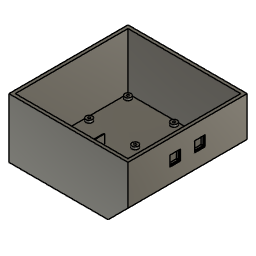
WeatherBox (Autodesk Fusion 360 design; units mm, degrees)
Autodesk Fusion 360 part; units mm, degrees
note: some values were not read from the file. Set by a fixed rule: which face or edge a step refers to.
sketch "Enclosure" plane through (0, 0, 0) normal (0, 0, 1) x (1, 0, 0)
  line L0 (0, 0) -> (150, 0)
  line L1 (150, 0) -> (150, 150)
  line L2 (150, 150) -> (0, 150)
  line L3 (0, 150) -> (0, 0)
  dimension "d1" = 150
  dimension "d2" = 150
  constraint horizontal L0
  constraint vertical L1
  constraint horizontal L2
  constraint vertical L3
  constraint coincident L0.start L3.end
  measures "d1" distance of L0.start L0.end
  measures "d2" distance of L0.start L2.end
extrude "Extrude1" add sketch "Enclosure" along normal blind 75 makes body 1
chamfer "Chamfer1" distance 25 angle 45 1 edges at (150, 75, 0) on bodies 1
shell "Shell1" thickness 4 removed faces 1 at (50, 100, 75) on bodies 1
sketch "Pi Mount" plane through (0, 0, 4) normal (0, 0, 1) x (-1, 0, 0)
  line L0 (-4, -146) -> (-4, -4)
  line L1 (-4, -4) -> (-123.3431, -4)
  line L2 (-123.3431, -146) -> (-4, -146)
  circle A0 centre (-9, -141) radius 4
  line L3 (-123.3431, -4) -> (-123.3431, -146)
  dimension "d13" = 8
  dimension "d39" = 5
  dimension "d40" = 5
  measures "d13" diameter of A0
  measures "d39" distance of L2 A0.centre
  measures "d40" distance of L0 A0.centre
extrude "Extrude2" add sketch "Pi Mount" along normal blind 3.1 contours A0 bodies 1
hole "Hole2" at (9, 141, 7.1) direction (0, 0, -1) diameter 2.9 depth 3.1 tip angle 180 bodies 1
pattern_linear "R-Pattern1" count 2 spacing 58 along (1, 0, 0) count 2 spacing 49 along (0, -1, 0) of "Extrude2", "Hole2"
sketch "Camera Holes" plane through (150, 0, 0) normal (1, 0, 0) x (0, 1, 0)
  line L0 (150, 25) -> (150, 75)
  line L1 (150, 75) -> (0, 75)
  line L2 (0, 75) -> (0, 25)
  line L3 (65, 44.45) -> (53.9, 44.45)
  line L4 (53.9, 44.45) -> (53.9, 55.55)
  line L5 (53.9, 55.55) -> (65, 55.55)
  line L6 (65, 55.55) -> (65, 44.45)
  line L7 (65, 44.45) -> (53.9, 55.55) construction
  line L8 (53.9, 44.45) -> (65, 55.55) construction
  line L9 (0, 50) -> (150, 50) construction
  line L10 (75, 75) -> (75, 0) construction
  line L11 (96.1, 44.45) -> (85, 55.55) construction
  line L12 (85, 44.45) -> (96.1, 55.55) construction
  line L13 (85, 44.45) -> (85, 55.55)
  line L14 (85, 55.55) -> (96.1, 55.55)
  line L15 (96.1, 55.55) -> (96.1, 44.45)
  line L16 (96.1, 44.45) -> (85, 44.45)
  line L17 (66, 43.45) -> (52.9, 43.45)
  line L18 (52.9, 43.45) -> (52.9, 56.55)
  line L19 (52.9, 56.55) -> (66, 56.55)
  line L20 (66, 56.55) -> (66, 43.45)
  line L21 (97.1, 43.45) -> (84, 43.45)
  line L22 (84, 43.45) -> (84, 56.55)
  line L23 (84, 56.55) -> (97.1, 56.55)
  line L24 (97.1, 56.55) -> (97.1, 43.45)
  line L25 (0, 25) -> (150, 25)
  point P0 (59.45, 50)
  point P1 (90.55, 50)
  dimension "d92" = 11.1
  dimension "d93" = 11.1
  dimension "d168" = 11.1
  dimension "d169" = 11.1
  dimension "d170" = 20
  dimension "d177" = -1
  dimension "d178" = -1
  constraint horizontal L3
  constraint perpendicular L3 L4
  constraint parallel L3 L5
  constraint parallel L4 L6
  constraint coincident L7 P0
  constraint coincident L8 P0
  constraint midpoint L2 L9.start
  constraint midpoint L0 L9.end
  constraint coincident P0 L9
  constraint midpoint L1 L10.start
  constraint horizontal L16
  constraint perpendicular L13 L16
  constraint parallel L14 L16
  constraint parallel L13 L15
  constraint coincident P1 L11
  constraint coincident P1 L12
  constraint symmetric L6 L10 L13
  constraint collinear L19 L23
  measures "d92" distance of L4.end L5.end
  measures "d93" distance of L3.end L4.end
  measures "d168" distance of L12.end L11.end
  measures "d169" distance of L12.start L11.end
  measures "d170" distance of L6 L13
extrude "Extrude6" cut sketch "Camera Holes" against normal up to surface (4 mm away) contours L3 L4 L5 L6 | L13 L14 L15 L16 bodies 1
extrude "Extrude10" cut sketch "Camera Holes" against normal blind 1.5875 contours L17 L18 L19 L20 | L21 L22 L23 L24 bodies 1
sketch "Camera Mounts" plane through (146, 0, 0) normal (-1, 0, 0) x (0, -1, 0)
  line L0 (-65, 44.45) -> (-65, 55.55)
  line L1 (-65, 55.55) -> (-53.9, 55.55)
  line L2 (-53.9, 55.55) -> (-53.9, 44.45)
  line L3 (-53.9, 44.45) -> (-65, 44.45)
  line L4 (-4, 26.6569) -> (-4, 75)
  line L5 (-4, 75) -> (-146, 75)
  line L6 (-146, 75) -> (-146, 26.6569)
  line L7 (-69.95, 62.6) -> (-48.95, 62.6) construction
  line L8 (-48.95, 62.6) -> (-48.95, 50.1) construction
  line L9 (-48.95, 50.1) -> (-69.95, 50.1) construction
  line L10 (-69.95, 50.1) -> (-69.95, 62.6) construction
  line L11 (-59.45, 55.55) -> (-59.45, 50) construction
  line L12 (-59.45, 50) -> (-53.9, 50) construction
  line L13 (-85, 44.45) -> (-96.1, 44.45)
  line L14 (-96.1, 44.45) -> (-96.1, 55.55)
  line L15 (-96.1, 55.55) -> (-85, 55.55)
  line L16 (-85, 55.55) -> (-85, 44.45)
  line L17 (-101.05, 62.6) -> (-80.05, 62.6) construction
  line L18 (-101.05, 50.1) -> (-101.05, 62.6) construction
  line L19 (-80.05, 50.1) -> (-101.05, 50.1) construction
  line L20 (-80.05, 62.6) -> (-80.05, 50.1) construction
  line L21 (-85, 50) -> (-90.55, 50) construction
  line L22 (-90.55, 50) -> (-90.55, 55.55) construction
  line L23 (-146, 26.6569) -> (-4, 26.6569)
  dimension "d131" = 21
  dimension "d132" = 12.5
  dimension "d173" = 21
  dimension "d174" = 12.5
  dimension "d176" = 0.1
  constraint horizontal L7
  constraint vertical L8
  constraint horizontal L9
  constraint vertical L10
  constraint midpoint L1 L11.start
  constraint perpendicular L1 L11
  constraint midpoint L2 L12.end
  constraint perpendicular L2 L12
  constraint horizontal L17
  constraint vertical L20
  constraint horizontal L19
  constraint vertical L18
  constraint midpoint L16 L21.start
  constraint midpoint L15 L22.end
  constraint perpendicular L15 L22
  constraint symmetric L18 L20 L22
  constraint collinear L9 L19
  measures "d131" distance of L7.start L7.end
  measures "d132" distance of L7.start L9.end
  measures "d173" distance of L17.start L17.end
  measures "d174" distance of L17.start L18.start
  measures "d176" distance of L19 L21
hole "Hole7" at (146, 48.95, 62.6) at (146, 69.95, 50.1) at (146, 80.05, 62.6) at (146, 101.05, 62.6) at (146, 101.05, 50.1) at (146, 80.05, 50.1) at (146, 69.95, 62.6) at (146, 48.95, 50.1) direction (1, 0, 0) diameter 2.9 depth 2 tip angle 180 bodies 1
sketch "Camera Posts" plane through (146, 0, 0) normal (-1, 0, 0) x (0, -1, 0)
  circle A0 centre (-101.05, 50.1) radius 1.45
  circle A1 centre (-80.05, 62.6) radius 1.45
  circle A2 centre (-48.95, 50.1) radius 1.45
  circle A3 centre (-69.95, 62.6) radius 1.45
  circle A4 centre (-48.95, 62.6) radius 1.45
  circle A5 centre (-69.95, 50.1) radius 1.45
  circle A6 centre (-101.05, 62.6) radius 1.45
  circle A7 centre (-80.05, 50.1) radius 1.45
  line L0 (-65, 44.45) -> (-65, 55.55)
  line L1 (-65, 55.55) -> (-53.9, 55.55)
  line L2 (-53.9, 55.55) -> (-53.9, 44.45)
  line L3 (-53.9, 44.45) -> (-65, 44.45)
  line L4 (-85, 44.45) -> (-96.1, 44.45)
  line L5 (-96.1, 44.45) -> (-96.1, 55.55)
  line L6 (-96.1, 55.55) -> (-85, 55.55)
  line L7 (-85, 55.55) -> (-85, 44.45)
  line L8 (-4, 26.6569) -> (-4, 75)
  line L9 (-4, 75) -> (-146, 75)
  line L10 (-146, 75) -> (-146, 26.6569)
  circle A8 centre (-101.05, 62.6) radius 3.95
  circle A9 centre (-80.05, 62.6) radius 3.95
  circle A10 centre (-101.05, 50.1) radius 3.95
  circle A11 centre (-80.05, 50.1) radius 3.95
  circle A12 centre (-69.95, 62.6) radius 3.95
  circle A13 centre (-48.95, 62.6) radius 3.95
  circle A14 centre (-48.95, 50.1) radius 3.95
  circle A15 centre (-69.95, 50.1) radius 3.95
  line L11 (-146, 26.6569) -> (-4, 26.6569)
  dimension "d193" = 2.5
  constraint equal A8 A10
  constraint equal A8 A11
  constraint equal A8 A9
  constraint equal A8 A12
  constraint equal A8 A15
  constraint equal A8 A14
  constraint equal A8 A13
extrude "Extrude11" add sketch "Camera Posts" along normal blind 7 contours A8 | A9 | A10 | A11 | A12 | A13 | A14 | A15 bodies 1
sketch "SPS30 Mount" plane through (0, 4, 0) normal (0, 1, 0) x (-1, 0, 0)
  line L0 (-4, 75) -> (-146, 75)
  line L1 (-123.3431, 4) -> (-4, 4)
  line L2 (-130, 64) -> (-83.15, 64)
  line L3 (-83.15, 64) -> (-83.15, 17.15)
  line L4 (-83.15, 17.15) -> (-130, 17.15)
  line L5 (-130, 17.15) -> (-130, 64)
  line L6 (-82.15, 16.15) -> (-131, 16.15)
  line L7 (-131, 16.15) -> (-131, 65)
  line L8 (-131, 65) -> (-82.15, 65)
  line L9 (-82.15, 65) -> (-82.15, 16.15)
  line L10 (-103.15, 17.15) -> (-103.15, 16.15)
  line L11 (-130, 17.15) -> (-130, 16.15)
  line L12 (-85.15, 64) -> (-85.15, 65)
  line L13 (-125, 64) -> (-125, 65)
  line L14 (-139.7177, 40.575) -> (-2.7177, 40.575) construction
  line L15 (-106.575, 64) -> (-106.575, 17.15) construction
  line L16 (-130, 40.575) -> (-83.15, 40.575) construction
  line L17 (-4, 4) -> (-4, 75)
  line L18 (-146, 75) -> (-146, 26.6569)
  line L19 (-104.15, 64) -> (-104.15, 75)
  line L20 (-104.15, 75) -> (-103.15, 75)
  line L21 (-103.15, 75) -> (-103.15, 64)
  line L22 (-104.15, 64) -> (-103.15, 64)
  line L23 (-78.15, 40.575) -> (-135, 40.575) construction
  circle A0 centre (-78.15, 40.575) radius 2.35
  circle A1 centre (-135, 40.575) radius 2.35
  circle A2 centre (-135, 40.575) radius 4.85
  circle A3 centre (-78.15, 40.575) radius 4.85
  line L24 (-78.15, 45.425) -> (-135, 45.425)
  line L25 (-135, 35.725) -> (-78.15, 35.725)
  line L26 (-146, 26.6569) -> (-123.3431, 4)
  dimension "d118" = 46.85
  dimension "d119" = 46.85
  dimension "d121" = -1
  dimension "d122" = 20
  dimension "d124" = 2
  dimension "d125" = 5
  dimension "d143" = 20
  dimension "d182" = 15
  dimension "d184" = 10
  dimension "d203" = 1
  dimension "d225" = 56.85
  dimension "d229" = 4.7
  dimension "d230" = 4.7
  dimension "d231" = 2.5
  dimension "d232" = 2.5
  constraint horizontal L2
  constraint vertical L3
  constraint horizontal L4
  constraint vertical L5
  constraint coincident L4 L10.start
  constraint coincident L6 L10.end
  constraint perpendicular L6 L10
  constraint coincident L6 L11.end
  constraint perpendicular L6 L11
  constraint coincident L2 L12.start
  constraint coincident L8 L12.end
  constraint perpendicular L8 L12
  constraint coincident L2 L13.start
  constraint coincident L8 L13.end
  constraint perpendicular L8 L13
  constraint midpoint L2 L15.start
  constraint midpoint L4 L15.end
  constraint midpoint L5 L16.start
  constraint midpoint L3 L16.end
  constraint collinear L14 L16
  constraint vertical L19
  constraint horizontal L20
  constraint vertical L21
  constraint coincident L0 L19.end
  constraint coincident L2 L19.start
  constraint coincident L2 L21.end
  constraint coincident L14 L23.start
  constraint perpendicular L15 L23
  constraint midpoint L15 L23
  constraint coincident L23.start A0.centre
  constraint coincident L23.end A1.centre
  constraint coincident A3 L24.start
  constraint coincident A2 L24.end
  constraint coincident A2 L25.start
  constraint coincident A3 L25.end
  constraint tangent A3 L24
  constraint tangent A3 L25
  constraint tangent A2 L25
  constraint tangent A2 L24
  measures "d118" distance of L2.start L4.end
  measures "d119" distance of L2.start L2.end
  measures "d122" distance of L3 L10
  measures "d124" distance of L3 L12
  measures "d125" distance of L5 L13
  measures "d143" distance of L3 L21
  measures "d182" distance of L7 L18
  measures "d184" distance of L0 L8
  measures "d203" distance of L21.end L19.start
  measures "d225" distance of L23.start L23.end
  measures "d229" diameter of A0
  measures "d230" diameter of A1
extrude "Extrude8" add sketch "SPS30 Mount" along normal blind 5 contours L2 L3 L8 L9 L12 L24 | L2 L5 L7 L8 L13 L24 | L9 A3 L24 | L3 L9 A3 L24 L25 | L5 L7 A2 L24 L25 | L7 A2 L24 | L9 A3 | L9 A3 | L7 A2 | L7 A2 | L9 A3 L25 | L3 L4 L6 L9 L10 L25 | L7 A2 L25 | L5 L6 L7 L11 L25 bodies 1
extrude "Extrude12" add sketch "SPS30 Mount" along normal blind 12.5 contours L0 L8 L19 L20 L21 | L2 L8 L19 L21 L22 bodies 1
fillet "Fillet1" radius 0.5 8 edges at (148, 53.9, 55.55) (148, 65, 44.45) (148, 65, 55.55) (148, 53.9, 44.45) (148, 96.1, 44.45) (148, 85, 44.45) (148, 85, 55.55) (148, 96.1, 55.55) on bodies 1
sketch "Wall STEMMA Mounts" plane through (0, 4, 0) normal (0, 1, 0) x (-1, 0, 0)
  line L0 (-85.15, 64) -> (-85.15, 65)
  line L1 (-85.15, 65) -> (-82.15, 65)
  line L2 (-82.15, 65) -> (-82.15, 45.425)
  line L3 (-82.15, 45.425) -> (-78.15, 45.425)
  arc A0 (-78.15, 35.725) -> (-78.15, 45.425) centre (-78.15, 40.575) ccw
  line L4 (-78.15, 35.725) -> (-82.15, 35.725)
  line L5 (-82.15, 35.725) -> (-82.15, 16.15)
  line L6 (-82.15, 16.15) -> (-103.15, 16.15)
  line L7 (-103.15, 16.15) -> (-103.15, 17.15)
  line L8 (-103.15, 17.15) -> (-83.15, 17.15)
  line L9 (-83.15, 17.15) -> (-83.15, 64)
  line L10 (-83.15, 64) -> (-85.15, 64)
  line L11 (-104.15, 75) -> (-146, 75)
  line L12 (-103.15, 75) -> (-103.15, 64)
  line L13 (-103.15, 64) -> (-104.15, 64)
  line L14 (-104.15, 64) -> (-104.15, 75)
  line L15 (-123.3431, 4) -> (-4, 4)
  line L16 (-131, 45.425) -> (-131, 65)
  line L17 (-131, 65) -> (-125, 65)
  line L18 (-125, 65) -> (-125, 64)
  line L19 (-125, 64) -> (-130, 64)
  line L20 (-130, 64) -> (-130, 16.15)
  line L21 (-130, 16.15) -> (-131, 16.15)
  line L22 (-131, 16.15) -> (-131, 35.725)
  line L23 (-131, 35.725) -> (-135, 35.725)
  arc A1 (-135, 45.425) -> (-135, 35.725) centre (-135, 40.575) ccw
  line L24 (-135, 45.425) -> (-131, 45.425)
  circle A2 centre (-16.5, 65) radius 1.45
  circle A3 centre (-16.5, 65) radius 3.95
  line L25 (-146, 75) -> (-146, 26.6569)
  line L26 (-4, 4) -> (-4, 75)
  line L27 (-4, 75) -> (-103.15, 75)
  line L28 (-146, 26.6569) -> (-123.3431, 4)
  dimension "d284" = 2.9
  dimension "d285" = 2.5
  dimension "d287" = 10
  measures "d284" diameter of A2
  measures "d287" distance of L11 A2.centre
extrude "Extrude19" add sketch "Wall STEMMA Mounts" along normal blind 3 contours A3 bodies 1
pattern_linear "R-Pattern7" count 2 spacing 12.7 along (1, 0, 0) count 2 spacing 20.32 along (0, 0, -1) of "Extrude19"
pattern_linear "R-Pattern8" count 2 spacing 25 along (1, 0, 0) of "Extrude19", "R-Pattern7"
sketch "Sketch1" plane through (0, 9, 0) normal (0, 1, 0) x (-1, 0, 0) in component "SPS Bar"
  circle A0 centre (-135, 40.575) radius 2.35
  line L0 (-130, 16.15) -> (-130, 64)
  line L1 (-130, 64) -> (-125, 64)
  line L2 (-125, 64) -> (-125, 65)
  line L3 (-125, 65) -> (-131, 65)
  line L4 (-131, 35.725) -> (-131, 16.15)
  arc A1 (-135, 45.425) -> (-135, 35.725) centre (-135, 40.575) ccw
  line L5 (-131, 16.15) -> (-130, 16.15)
  circle A2 centre (-78.15, 40.575) radius 2.35
  line L6 (-82.15, 16.15) -> (-82.15, 35.725)
  arc A3 (-78.15, 35.725) -> (-78.15, 45.425) centre (-78.15, 40.575) ccw
  line L7 (-82.15, 65) -> (-85.15, 65)
  line L8 (-85.15, 65) -> (-85.15, 64)
  line L9 (-85.15, 64) -> (-83.15, 64)
  line L10 (-83.15, 64) -> (-83.15, 17.15)
  line L11 (-83.15, 17.15) -> (-103.15, 17.15)
  line L12 (-103.15, 17.15) -> (-103.15, 16.15)
  line L13 (-103.15, 16.15) -> (-82.15, 16.15)
  line L14 (-78.15, 45.425) -> (-135, 45.425)
  line L15 (-135, 35.725) -> (-78.15, 35.725)
  circle A4 centre (-78.15, 40.575) radius 1.5
  circle A5 centre (-135, 40.575) radius 1.5
  line L16 (-131, 45.425) -> (-135, 45.425)
  line L17 (-135, 35.725) -> (-131, 35.725)
  line L18 (-131, 65) -> (-131, 45.425)
  line L19 (-82.15, 35.725) -> (-78.15, 35.725)
  line L20 (-78.15, 45.425) -> (-82.15, 45.425)
  line L21 (-82.15, 45.425) -> (-82.15, 65)
  dimension "d269" = 3
  constraint coincident A3 L14.start
  constraint coincident A1 L14.end
  constraint tangent A3 L14
  constraint tangent A1 L14
  constraint coincident A1 L15.start
  constraint coincident A3 L15.end
  constraint tangent A1 L15
  constraint tangent A3 L15
  constraint concentric A2 A4
  constraint concentric A0 A5
  constraint equal A4 A5
  measures "d269" diameter of A4
extrude "Extrude1'" add sketch "Sketch1" along normal blind 3 separate body contours A0 | L0 A1 L14 L15 L16 L17 | L0 L10 L14 L15 | A3 L10 L14 L15 L19 L20 | A2 makes body 2 in component "SPS Bar"
sketch "Sketch2" plane through (0, 9, 0) normal (0, -1, 0) x (1, 0, 0) in component "SPS Bar"
  circle A0 centre (78.15, 40.575) radius 1.5
  circle A1 centre (135, 40.575) radius 1.5
  line L0 (78.15, 35.725) -> (135, 35.725)
  arc A2 (135, 35.725) -> (135, 45.425) centre (135, 40.575) ccw
  line L1 (135, 45.425) -> (78.15, 45.425)
  arc A3 (78.15, 45.425) -> (78.15, 35.725) centre (78.15, 40.575) ccw
  line L2 (78.8, 45.425) -> (120, 45.425)
  line L3 (120, 45.425) -> (120, 35.725)
  line L4 (120, 35.725) -> (78.8, 35.725)
  line L5 (78.8, 35.725) -> (78.8, 45.425)
  constraint horizontal L2
  constraint vertical L3
  constraint horizontal L4
  constraint vertical L5
  constraint coincident L0 L3.end
  constraint coincident L1 L2.start
sketch "Bar Height" plane through (0, 12, 0) normal (0, 1, 0) x (-1, 0, 0) in component "SPS Bar"
  circle A0 centre (-78.15, 40.575) radius 1.5
  circle A1 centre (-135, 40.575) radius 1.5
  line L0 (-135, 35.725) -> (-78.15, 35.725)
  arc A2 (-78.15, 35.725) -> (-78.15, 45.425) centre (-78.15, 40.575) ccw
  line L1 (-78.15, 45.425) -> (-135, 45.425)
  arc A3 (-135, 45.425) -> (-135, 35.725) centre (-135, 40.575) ccw
  line L2 (-83.15, 64) -> (-83.15, 17.15)
  line L3 (-130, 16.15) -> (-130, 64)
  line L4 (-81.15, 64) -> (-81.15, 22.8)
  line L5 (-132, 21.8) -> (-132, 64)
  dimension "d272" = -2
  dimension "d273" = -2
extrude "Extrude3" add sketch "Bar Height" along normal blind 12 contours L0 L1 L3 L5 | L0 L1 L2 L3 | L0 L1 L2 L4 bodies 2 in component "SPS Bar"
sketch "SPS Cut" plane through (0, 9, 0) normal (0, -1, 0) x (1, 0, 0) in component "SPS Bar"
  circle A0 centre (78.15, 40.575) radius 1.5
  circle A1 centre (135, 40.575) radius 1.5
  line L0 (78.15, 35.725) -> (135, 35.725)
  arc A2 (135, 35.725) -> (135, 45.425) centre (135, 40.575) ccw
  line L1 (135, 45.425) -> (78.15, 45.425)
  arc A3 (78.15, 45.425) -> (78.15, 35.725) centre (78.15, 40.575) ccw
  line L2 (130, 16.15) -> (130, 64)
  line L3 (83.15, 64) -> (83.15, 17.15)
extrude "Extrude4" cut sketch "SPS Cut" against normal blind 12.85 contours L0 L1 L2 L3 bodies 2 in component "SPS Bar"
fillet "Fillet1'" radius 3 4 edges at (81.15, 12, 40.575) (81.15, 24, 40.575) (132, 24, 40.575) (132, 12, 40.575) on bodies 2 in component "SPS Bar"
sketch "Angled STEMMA Mounts" plane through (59.6716, 0, -59.6716) normal (-0.707107, 0, 0.707107) x (0, -1, 0)
  line L0 (-146, 90.0452) -> (-4, 90.0452)
  line L1 (-4, 90.0452) -> (-4, 122.0868)
  line L2 (-4, 122.0868) -> (-146, 122.0868)
  line L3 (-146, 122.0868) -> (-146, 90.0452)
  line L4 (-75, 122.0868) -> (-75, 90.0452) construction
  circle A0 centre (-80, 116.226) radius 1.45
  circle A1 centre (-80, 116.226) radius 2.95
  circle A2 centre (-92.7, 116.226) radius 1.45
  circle A3 centre (-92.7, 116.226) radius 2.95
  circle A4 centre (-80, 95.906) radius 1.45
  circle A5 centre (-80, 95.906) radius 2.95
  circle A6 centre (-92.7, 95.906) radius 1.45
  circle A7 centre (-92.7, 95.906) radius 2.95
  line L5 (-75, 106.066) -> (-66.9778, 106.066) construction
  circle A8 centre (-70, 116.226) radius 1.45
  circle A9 centre (-70, 116.226) radius 2.95
  circle A10 centre (-70, 95.906) radius 1.45
  circle A11 centre (-70, 95.906) radius 2.95
  circle A12 centre (-57.3, 95.906) radius 1.45
  circle A13 centre (-57.3, 95.906) radius 2.95
  circle A14 centre (-57.3, 116.226) radius 1.45
  circle A15 centre (-57.3, 116.226) radius 2.95
  dimension "d299" = 2.9
  dimension "d300" = 1.5
  dimension "d303" = 12.7
  dimension "d304" = 20.32
  dimension "d305" = 10
  constraint midpoint L2 L4.start
  constraint coincident L0 L4.end
  constraint perpendicular L0 L4
  constraint midpoint L4 L5.start
  constraint perpendicular L4 L5
  constraint symmetric A0 A4 L5
  constraint symmetric L4 A0 A8
  constraint symmetric L4 A1 A9
  constraint symmetric L4 A2 A14
  constraint symmetric L4 A3 A15
  constraint symmetric L4 A4 A10
  constraint symmetric L4 A5 A11
  constraint symmetric L4 A6 A12
  constraint symmetric L4 A7 A13
  measures "d299" diameter of A0
  measures "d305" distance of A0.centre A8.centre
extrude "Extrude20" add sketch "Angled STEMMA Mounts" along normal blind 3 contours A1 | A3 | A5 | A7 | A9 | A11 | A13 | A15 bodies 1
sketch "Light Sensors Hole" plane through (62.5, 0, -62.5) normal (0.707107, 0, -0.707107) x (0, 1, 0)
  line L0 (150, 88.3883) -> (150, 123.7437)
  line L1 (150, 123.7437) -> (0, 123.7437)
  line L2 (0, 123.7437) -> (0, 88.3883)
  line L3 (0, 88.3883) -> (150, 88.3883)
  circle A0 centre (92.7, 116.226) radius 2.95
  circle A1 centre (57.3, 116.226) radius 2.95
  circle A2 centre (57.3, 95.906) radius 2.95
  circle A3 centre (92.7, 95.906) radius 2.95
  line L4 (54.35, 113.276) -> (95.65, 113.276)
  line L5 (95.65, 113.276) -> (95.65, 98.856)
  line L6 (95.65, 98.856) -> (54.35, 98.856)
  line L7 (54.35, 98.856) -> (54.35, 113.276)
  line L8 (96.65, 97.856) -> (53.35, 97.856)
  line L9 (53.35, 97.856) -> (53.35, 114.276)
  line L10 (53.35, 114.276) -> (96.65, 114.276)
  line L11 (96.65, 114.276) -> (96.65, 97.856)
  circle A4 centre (92.7, 116.226) radius 2.95
  circle A5 centre (57.3, 116.226) radius 2.95
  circle A6 centre (57.3, 95.906) radius 2.95
  circle A7 centre (92.7, 95.906) radius 2.95
  dimension "d318" = -1
  constraint horizontal L4
  constraint vertical L5
  constraint horizontal L6
  constraint vertical L7
  constraint tangent L7 A5
  constraint tangent L5 A4
  constraint tangent L4 A5
  constraint tangent A2 L6
extrude "Extrude25" cut sketch "Light Sensors Hole" against normal up to surface (4 mm away) contours L4 L5 L6 L7 bodies 1
extrude "Extrude26" cut sketch "Light Sensors Hole" against normal blind 1.5875 contours A0 L10 A4 | A0 A1 L4 L10 A4 A5 | A0 A3 L4 L5 L6 L8 L10 L11 A4 A7 | A1 L10 A5 | A1 A2 L4 L6 L7 L8 L9 L10 A5 A6 | A3 L8 A7 | A2 A3 L6 L8 A6 A7 | A2 L8 A6 picked at (92.0611, 114.1785) picked at (56.6611, 114.1785) picked at (92.4624, 98.2771) picked at (57.2731, 98.4572) bodies 1
component "SPS Bar" placed x (1, 0, 0) y (0, 1, 0) z (0, 0, 1) at (0, 0, 0)
equation "PI_MOUNT_HOLE_SEP_W = 58 mm" comment "Distance between Pi mount holes (parallel GPIO)"
equation "PI_MOUNT_HOLE_SEP_H = 49 mm" comment "Distance between Pi mount holes (perpendicular GPIO)"
equation "d14 = PI_BOTTOM_CLEARANCE"
equation "PI_BOTTOM_CLEARANCE = 3.1 mm" comment "Height of cooler mount pins from bottom surface of Pi"
equation "d17 = PI_BOTTOM_CLEARANCE"
equation "d22 = PI_MOUNT_HOLE_SEP_W"
equation "d23 = PI_MOUNT_HOLE_SEP_H"
equation "LTR390_MOUNT_HOLE_SEP_W = 0.8 mm"
equation "LTR390_MOUNT_HOLE_SEP_H = 0.5 mm"
equation "LTR390_W = 1 mm"
equation "LTR390_H = 0.7 mm"
equation "STEMMA_W = 25.4 mm" comment "STEMMA Board Width"
equation "STEMMA_H = 17.78 mm" comment "STEMMA Board Length"
equation "STEMMA_MOUNT_HOLE_SEP_W = 20.32 mm" comment "STEMMA Mount Hole Separation Width"
equation "STEMMA_MOUNT_HOLE_SEP_H = 12.7 mm" comment "STEMMA Mount Hole Separation Length"
equation "AS3935_HOLE = 3 mm"
equation "AS3935_W = 26 mm"
equation "d92 = CAM_W + 0.2 mm"
equation "d93 = CAM_W + 0.2 mm"
equation "ARDUCAM_COVER_W = 31.5 mm"
equation "ARDUCAM_COVER_H = 30.5 mm"
equation "CAM_W = 10.9 mm"
equation "SPS30_EXHAUST_W = 14.8 mm"
equation "SPS30_EXHAUST_H = 4.75 mm"
equation "SPS30_INTAKE_W = 6.6 mm"
equation "SPS30_INTAKE_H = 3.5 mm"
equation "SPS30_W = 40.5 mm"
equation "SPS30_TOP_INTAKE_W = 10 mm"
equation "SPS30_TOP_INTAKE_H = 1.2 mm"
equation "d118 = SPS30_W + ( 0.125 in * 2 )"
equation "d119 = SPS30_W + ( 0.125 in * 2 )"
equation "AS3935_HOLE_SPACING = 30.5 mm"
equation "d168 = CAM_W + 0.2 mm"
equation "d169 = CAM_W + 0.2 mm"
equation "d179 = -CAMERA_PROTECTOR_THICKNESS"
equation "CAMERA_PROTECTOR_THICKNESS = 0.0625 in"
equation "d225 = d119 + 10 mm"
equation "d276 = -12.5 mm - ( 0.125 in * 2 ) + 5 mm + 1 mm"
equation "d292 = STEMMA_MOUNT_HOLE_SEP_H"
equation "d293 = -STEMMA_MOUNT_HOLE_SEP_W"
equation "d303 = STEMMA_MOUNT_HOLE_SEP_H"
equation "d304 = STEMMA_MOUNT_HOLE_SEP_W"
equation "d321 = -CAMERA_PROTECTOR_THICKNESS"
named bodies: "Enclosure"
